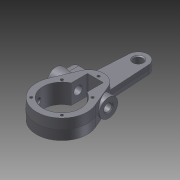
# Autodesk Inventor part: Piesa - 002 Lever
Saved by Autodesk Inventor 2011 SP2 (Build 150309200, 309)
## iProperties
Created: 2023-05-08
Part Number: Piesa - 002 Lever
Document SubType Name: Modeling
Designer: utilizator
Density: 1 g/cm^3
Author: utilizator
Autodesk Inventor part; units mm, degrees
ref_plane "XY Plane" through (0, 0, 0) normal (0, 0, 1) x (1, 0, 0)
sketch "Sketch1" plane through (0, 0, 0) normal (0, 0, 1) x (1, 0, 0)
  arc A0 (-38.7386, 16.2273) -> (38.7682, 16.1562) centre (0, 0) ccw
  line L0 (-38.7386, 16.2273) -> (-23.0587, 53.6591)
  arc A1 (23.0409, 53.7013) -> (-23.0587, 53.6591) centre (0, 44) ccw
  arc A2 (38.7682, 16.1562) -> (23.0409, 53.7013) centre (-10213.9791, -4256.5631) ccw
  dimension "d0" = 42
  dimension "d1" = 25
  dimension "d2" = 44
  constraints: 6 point on circle, 4 tangent, 3 centre point, 2 end point, 1 coincident, 1 vertical alignment
  measures "d0" radius of A0
  measures "d1" radius of A1
  measures "d2" distance of point (0, 0) A1.centre
extrude "Extrusion1" add sketch "Sketch1" along normal mid plane 32 draft -2
sketch "Sketch2" plane through (0, 0, 0) normal (0, 0, 1) x (1, 0, 0)
  line L0 (-20.9841, 44) -> (20.9841, 44)
  arc A0 (15.9702, 125.9768) -> (-15.9702, 125.9768) centre (0, 125) ccw
  line L1 (-15.9702, 125.9768) -> (-20.9841, 44)
  line L2 (15.9702, 125.9768) -> (20.9841, 44)
  arc A1 (22.526, 53.4845) -> (-22.5433, 53.4432) centre (0, 44) ccw construction
  point P0 (0, 0)
  dimension "d5" = 16
  dimension "d6" = 125
  dimension "d7" = 7
  constraints: 6 end point, 2 point on circle, 2 tangent, 1 centre point, 1 coincident, 1 horizontal, 1 midpoint, 1 vertical alignment
  measures "d5" radius of A0
  measures "d6" distance of point (0, 0) A0.centre
  measures "d7" angle of L2 L1
extrude "Extrusion2" add sketch "Sketch2" along normal mid plane 14 draft -2
ref_plane "Work Plane1" through (37, 0, 0) normal (1, 0, 0) x (0, 1, 0)
sketch "Sketch3" plane through (37, 0, 0) normal (1, 0, 0) x (0, 1, 0)
  circle A0 centre (39.5, 0) radius 15
  point P0 (0, 0)
  dimension "d11" = 15
  dimension "d12" = 39.5
  constraints: 1 centre point, 1 horizontal alignment
  measures "d11" radius of A0
  measures "d12" distance of point (0, 0) A0.centre
extrude "Extrusion3" add sketch "Sketch3" against normal blind 86
sketch "Sketch4" plane through (0, 0, 16) normal (0, 0, 1) x (1, 0, 0)
  arc A0 (-38.2232, 16.0114) -> (38.2525, 15.9413) centre (0, 0) ccw projected
  circle A1 centre (0, 0) radius 31
  line L0 (-13, 0) -> (13, 0)
  line L1 (13, 0) -> (13, 55)
  line L2 (13, 55) -> (-13, 55)
  line L3 (-13, 55) -> (-13, 0)
  dimension "d15" = 31
  dimension "d16" = 26
  dimension "d17" = 55
  constraints: 8 end point, 2 coincident, 2 parallel, 1 centre point, 1 horizontal, 1 midpoint, 1 perpendicular
  measures "d15" radius of A1
  measures "d16" distance between parallel lines of L1 L3
  measures "d17" distance from line of A0.centre L2
extrude "Extrusion4" cut sketch "Sketch4" against normal through all
fillet "Fillet1" radius 1 1 edges at (-13, 55, 0)
fillet "Fillet2" radius 1 1 edges at (13, 55, 0)
ref_plane "Work Plane2" through (0, 60.5, 0) normal (0, 1, 0) x (-1, 0, 0)
sketch "Sketch5" plane through (0, 60.5, 0) normal (0, 1, 0) x (-1, 0, 0)
  line L0 (13, -16) -> (13, 16) projected
  line L1 (13, -14) -> (33, -14)
  arc A0 (33, -14) -> (33, 14) centre (33, 0) ccw
  line L2 (33, 14) -> (13, 14)
  line L3 (13, 14) -> (13, -14)
  point P0 (0, 0)
  point P1 (13, 0)
  dimension "d23" = 33
  dimension "d24" = 14
  constraints: 6 end point, 2 midpoint, 2 point on circle, 2 tangent, 1 centre point, 1 collinear, 1 parallel, 1 perpendicular
  measures "d23" distance of point (0, 0) A0.centre
  measures "d24" radius of A0
extrude "Extrusion5" add sketch "Sketch5" against normal up to surface
hole "Hole1" at (37, 39.5, 0) direction (-1, 0, 0) diameter 13 end up to surface
hole "Hole2" at (-49, 39.5, 0) direction (1, 0, 0) diameter 13.8 end up to surface
hole "Hole3" at (-33, 60.5, 0) direction (0, -1, 0) diameter 8.917 end up to surface thread size "M10x1" class "6H" standard "ISO Metric profile"
hole "Hole4" at (0, 125, 7) direction (0, 0, -1) diameter 15 end through all
sketch "Sketch6" plane through (0, 0, 16) normal (0, 0, 1) x (1, 0, 0)
  arc A0 (-13, 28.1425) -> (13, 28.1425) centre (0, 0) ccw projected
  arc A1 (-38.2232, 16.0114) -> (38.2525, 15.9413) centre (0, 0) ccw projected
  line L0 (-12265.1749, 0) -> (2093.1958, 0) projected
  line L1 (-25.1023, 25.1023) -> (0, 0) construction
  point P0 (0, 60)
  point P1 (-25.1023, -25.1023)
  point P2 (25.1023, -25.1023)
  point P3 (25.1023, 25.1023)
  dimension "d64" = 45
  dimension "d65" = 35.5
  dimension "d66" = 60
  dimension "d69" = 360
  constraints: 2 end point, 1 vertical alignment, 5 other
  measures "d64" angle of L0 L1
  measures "d65" distance of L1.start L1.end
  measures "d66" distance of A0.centre point (0, 60)
hole "Hole5" at (0, 60, 16) at (-25.1023, 25.1023, 16) at (-25.1023, -25.1023, 16) at (25.1023, -25.1023, 16) at (25.1023, 25.1023, 16) direction (0, 0, -1) diameter 4.3 end through all
sketch "Sketch7" plane through (0, 0, 0) normal (0, 0, 1) x (1, 0, 0)
  line L0 (0, 0) -> (-53.4675, -14.3266)
  line L1 (-71.2228, 0) -> (60.8705, 0) projected
  dimension "d78" = 15
  constraints: 2 end point
  measures "d78" angle of L1 L0
hole "Hole6" at (-40.5689, -10.8704, 0) direction (0.9659258, 0.258819, 0) diameter 8.917 end up to surface thread size "M10x1" class "6H" standard "ISO Metric profile"
chamfer "Chamfer1" distance 1.5 angle 45 2 edges at (0, 132.5, 7) (0, 132.5, -7)
chamfer "Chamfer2" distance 1.5 angle 45 3 edges at (-33, 60.5, -4.4585) (37, 39.5, 6.5) (-49, 39.5, -6.9)
body "Solid1"
